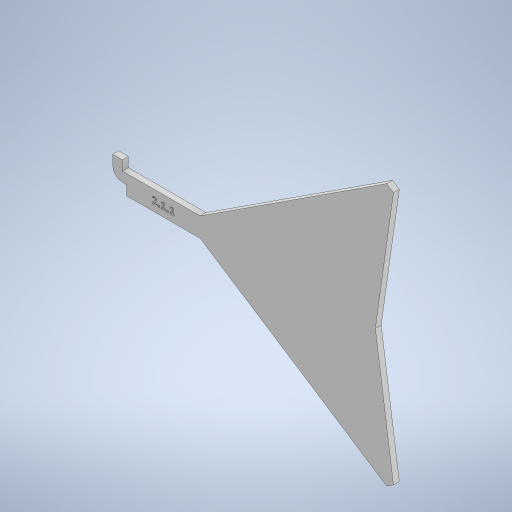
# Autodesk Inventor part: WindFinAlt
Saved by Autodesk Inventor 2024.3 (Build 283343000, 343)
## iProperties
Created: 2025-01-27
Part Number: WindFinAlt
Material: Generisch
Document SubType Name: Modeling
Designer: Maximilian Hock
Density: 1 g/cm^3
Appearance: Vorgabe
Author: Maximilian Hock
## iProperties of the stored document WindFinAlt_3D-Druck.ipt
Created: 2025-01-27
Part Number: WindFinAlt_3D-Druck
Material: Generisch
Document SubType Name: Modeling
Designer: Maximilian Hock
Density: 1 g/cm^3
Appearance: Vorgabe
Author: Maximilian Hock
Autodesk Inventor part; units mm, degrees
ref_plane "YZ Plane" through (0, 0, 0) normal (1, 0, 0) x (0, 1, 0)
ref_plane "XZ Plane" through (0, 0, 0) normal (0, 1, 0) x (-1, 0, 0)
ref_plane "XY Plane" through (0, 0, 0) normal (0, 0, 1) x (1, 0, 0)
sketch "Skizze1" plane through (0, 0, 0) normal (0, 1, 0) x (-1, 0, 0)
  line L0 (0, 0) -> (0, 5)
  line L1 (0, 5) -> (5, 5)
  line L2 (5, 5) -> (5, 0)
  line L3 (0, 0) -> (-40, 0)
  line L4 (-2, -5) -> (-2, -10)
  line L5 (-140, -75) -> (-130, -5)
  line L6 (-130, -5) -> (-140, 65)
  line L7 (-140, 65) -> (-40, 0)
  line L8 (0, -5) -> (-2, -5)
  line L9 (-2, -10) -> (-40, -10)
  line L10 (-40, -10) -> (-140, -75)
  line L11 (-40, -10) -> (-40, 0)
  arc A0 (0, -5) -> (5, 0) centre (0, 0) ccw
  point P0 (-40, -5)
  dimension "d2" = 100
  dimension "d3" = 5
  dimension "d4" = 140
  dimension "d5" = 10
  dimension "d6" = 140
  dimension "d7" = 2
  constraints: 24 end point, 4 equal length, 3 horizontal, 3 vertical, 2 perpendicular, 2 point on circle, 2 tangent, 1 centre point, 1 coincident, 1 horizontal alignment, 1 midpoint, 1 point on line
  measures "d2" horizontal distance of L6.end L3.end
  measures "d3" distance of L4.start L4.end
  measures "d4" distance of L5.start L6.end
  measures "d5" horizontal distance of L6.end L5.end
  measures "d6" horizontal distance of L6.end L0.start
  measures "d7" distance between parallel lines of L4 L0
extrude "Extrusion1" add sketch "Skizze1" along normal blind 3
chamfer "Fasen1" distance 5 angle 45 2 edges at (140, 1.5, 65) (140, 1.5, -75)
sketch "Skizze2" plane through (0, 0, 0) normal (0, -1, 0) x (1, 0, 0)
  line L0 (2, 0) -> (40, 0) construction
  line L1 (40, 0) -> (40, -10) construction
  line L2 (40, -10) -> (2, -10) construction
  line L3 (2, -10) -> (2, 0) construction
  line L4 (17.8248, -6.784) -> (15.2522, -6.784)
  line L5 (15.2522, -6.784) -> (15.2522, -6.2139)
  spline S0 degree 2 poles (15.2522, -6.2139) (15.5784, -5.953) (16.1003, -5.4935) (16.296, -5.2865) knots 0 0 0 1 2 2 2
  spline S1 degree 2 poles (16.296, -5.2865) (16.5541, -5.017) (16.7838, -4.6058) (16.7838, -4.3902) knots 0 0 0 1 2 2 2
  spline S2 degree 2 poles (16.7838, -4.3902) (16.7838, -4.1463) (16.4917, -3.8853) (16.2308, -3.8853) knots 0 0 0 1 2 2 2
  spline S3 degree 2 poles (16.2308, -3.8853) (16.0974, -3.8853) (15.8592, -3.9506) (15.7372, -4.0016) knots 0 0 0 1 2 2 2
  spline S4 degree 2 poles (15.7372, -4.0016) (15.6181, -4.0555) (15.4479, -4.169) (15.4054, -4.1973) knots 0 0 0 1 2 2 2
  line L6 (15.4054, -4.1973) -> (15.3373, -4.1973)
  line L7 (15.3373, -4.1973) -> (15.3373, -3.4344)
  spline S5 degree 2 poles (15.3373, -3.4344) (15.4848, -3.3635) (16.1145, -3.216) (16.4066, -3.216) knots 0 0 0 1 2 2 2
  spline S6 degree 2 poles (16.4066, -3.216) (17.0306, -3.216) (17.6716, -3.7719) (17.6716, -4.2739) knots 0 0 0 1 2 2 2
  spline S7 degree 2 poles (17.6716, -4.2739) (17.6716, -4.5831) (17.3795, -5.1787) (17.0419, -5.519) knots 0 0 0 1 2 2 2
  spline S8 degree 2 poles (17.0419, -5.519) (16.8292, -5.7289) (16.4293, -6.0551) (16.3414, -6.1232) knots 0 0 0 1 2 2 2
  line L8 (16.3414, -6.1232) -> (17.8248, -6.1232)
  line L9 (17.8248, -6.1232) -> (17.8248, -6.784)
  line L10 (19.1295, -6.784) -> (18.2984, -6.784)
  line L11 (18.2984, -6.784) -> (18.2984, -5.8594)
  line L12 (18.2984, -5.8594) -> (19.1295, -5.8594)
  line L13 (19.1295, -5.8594) -> (19.1295, -6.784)
  line L14 (22.238, -6.784) -> (19.9265, -6.784)
  line L15 (19.9265, -6.784) -> (19.9265, -6.1742)
  line L16 (19.9265, -6.1742) -> (20.6639, -6.1742)
  line L17 (20.6639, -6.1742) -> (20.6639, -4.3221)
  line L18 (20.6639, -4.3221) -> (19.9265, -4.3221)
  line L19 (19.9265, -4.3221) -> (19.9265, -3.752)
  spline S9 degree 2 poles (19.9265, -3.752) (20.0881, -3.752) (20.4086, -3.7095) (20.5051, -3.6641) knots 0 0 0 1 2 2 2
  spline S10 degree 2 poles (20.5051, -3.6641) (20.6157, -3.6074) (20.7405, -3.4173) (20.7518, -3.2755) knots 0 0 0 1 2 2 2
  line L20 (20.7518, -3.2755) -> (21.5176, -3.2755)
  line L21 (21.5176, -3.2755) -> (21.5176, -6.1742)
  line L22 (21.5176, -6.1742) -> (22.238, -6.1742)
  line L23 (22.238, -6.1742) -> (22.238, -6.784)
  line L24 (23.6987, -6.784) -> (22.8677, -6.784)
  line L25 (22.8677, -6.784) -> (22.8677, -5.8594)
  line L26 (22.8677, -5.8594) -> (23.6987, -5.8594)
  line L27 (23.6987, -5.8594) -> (23.6987, -6.784)
  line L28 (26.8073, -6.784) -> (24.4957, -6.784)
  line L29 (24.4957, -6.784) -> (24.4957, -6.1742)
  line L30 (24.4957, -6.1742) -> (25.2332, -6.1742)
  line L31 (25.2332, -6.1742) -> (25.2332, -4.3221)
  line L32 (25.2332, -4.3221) -> (24.4957, -4.3221)
  line L33 (24.4957, -4.3221) -> (24.4957, -3.752)
  spline S11 degree 2 poles (24.4957, -3.752) (24.6574, -3.752) (24.9779, -3.7095) (25.0744, -3.6641) knots 0 0 0 1 2 2 2
  spline S12 degree 2 poles (25.0744, -3.6641) (25.185, -3.6074) (25.3098, -3.4173) (25.3211, -3.2755) knots 0 0 0 1 2 2 2
  line L34 (25.3211, -3.2755) -> (26.0869, -3.2755)
  line L35 (26.0869, -3.2755) -> (26.0869, -6.1742)
  line L36 (26.0869, -6.1742) -> (26.8073, -6.1742)
  line L37 (26.8073, -6.1742) -> (26.8073, -6.784)
  point P0 (0, 0)
  point P1 (2, -10)
  constraints: 2 coincident, 2 other
emboss "Prägen1" sketch "Skizze2" operation cut depth 0.5 direction (0, 1, 0)
equation "\"d0\" = FinThickness"
equation "\"FinThickness\" = 3"
